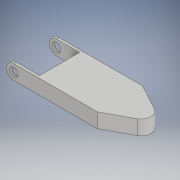
# Autodesk Inventor part: TIBIA
Saved by Autodesk Inventor 2017 (Build 210142000, 142)
## iProperties
Created: 2017-09-24
Part Number: TIBIA
Material: Generic
Document SubType Name: Modeling
Designer: Alexander Miller
Density: 1 g/cm^3
Appearance: Default
Author: Alexander Miller
Autodesk Inventor part; units mm, degrees
ref_plane "YZ Plane" through (0, 0, 0) normal (1, 0, 0) x (0, 1, 0)
ref_plane "XZ Plane" through (0, 0, 0) normal (0, 1, 0) x (-1, 0, 0)
ref_plane "XY Plane" through (0, 0, 0) normal (0, 0, 1) x (1, 0, 0)
sketch "Sketch1" plane through (0, 0, 0) normal (0, 1, 0) x (-1, 0, 0)
  line L0 (18.5, -50) -> (-18.5, -50) construction
  line L1 (-18.5, -50) -> (-18.5, 50) construction
  line L2 (-18.5, 50) -> (18.5, 50) construction
  line L3 (18.5, 50) -> (18.5, -50) construction
  line L4 (16.5, -50) -> (16.5, -25)
  line L5 (16.5, -25) -> (-16.5, -25)
  line L6 (-16.5, -25) -> (-16.5, -50)
  line L7 (-16.5, -50) -> (-18.5, -50)
  line L8 (-18.5, -50) -> (-18.5, 24.5296)
  line L9 (-18.5, 24.5296) -> (-6.9662, 45.8484)
  line L10 (-6.9662, 45.8484) -> (6.9662, 45.8484) construction
  line L11 (6.9662, 45.8484) -> (18.5, 24.5296)
  line L12 (18.5, 24.5296) -> (18.5, -50)
  line L13 (18.5, -50) -> (16.5, -50)
  arc A0 (6.9662, 45.8484) -> (-6.9662, 45.8484) centre (0, 42.0796) ccw
  point P0 (0, 0)
  point P1 (0, -50)
  point P2 (18.5, 0)
  point P3 (0, -25)
  point P4 (0, 45.8484)
  dimension "d0" = 100
  dimension "d1" = 37
  dimension "d2" = 25
  dimension "d3" = 2
  constraints: 28 end point, 5 collinear, 5 perpendicular, 4 midpoint, 3 parallel, 3 tangent, 3 vertical alignment, 2 point on circle, 1 centre point, 1 horizontal, 1 horizontal alignment, 1 point on line, 1 vertical
  measures "d0" distance of L2.end L0.start
  measures "d1" distance of L0.start L0.end
  measures "d2" distance between parallel lines of L5 L0
  measures "d3" distance between parallel lines of L4 L3
extrude "Extrusion1" add sketch "Sketch1" along normal blind 12
full round fillet "Fillet1" first side at (5.5, 12, 8.0197) centre faces at (17.1667, 4, -50) second side at (5.5, 0, 8.0197)
full round fillet "Fillet2" first side at (5.5, 0, 8.0197) centre faces at (-17.8333, 4, -50) second side at (5.5, 12, 8.0197)
sketch "Sketch2" plane through (-18.5, 0, 24.5296) normal (-1, 0, 0) x (0, 0, 1)
  circle A0 centre (-68.5296, 6) radius 3.5
  arc A1 (-68.5296, 12) -> (-68.5296, 0) centre (-68.5296, 6) ccw projected
  point P0 (-24.5296, 0)
  dimension "d6" = 7
  constraints: 1 centre point, 1 concentric
  measures "d6" diameter of A0
extrude "Extrusion2" cut sketch "Sketch2" against normal up to surface (2 mm away)
sketch "Sketch3" plane through (18.5, 0, 24.5296) normal (1, 0, 0) x (0, 0, -1)
  circle A0 centre (68.5296, 6) radius 3.625
  arc A1 (68.5296, 0) -> (68.5296, 12) centre (68.5296, 6) ccw projected
  point P0 (24.5296, 0)
  dimension "d9" = 7.25
  constraints: 1 centre point, 1 concentric
  measures "d9" diameter of A0
extrude "Extrusion3" cut sketch "Sketch3" against normal up to surface (2 mm away)
equation "\"d4\" = servo_B"
equation "\"d6\" = bearing_A"
equation "\"d7\" = servo_B"
equation "\"d9\" = servo_hat_A"
equation "\"d10\" = servo_B"
equation "\"servo_B\" = 12"
equation "\"bearing_A\" = 7"
equation "\"servo_hat_A\" = 7.25"
body "Solid1"
